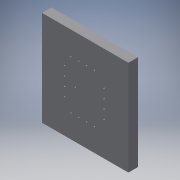
# Autodesk Inventor part: Trasera
Saved by Autodesk Inventor 2017 (Build 210142000, 142)
## iProperties
Created: 2021-02-12
Part Number: Trasera
Material: Generic
Document SubType Name: Modeling
Designer: USUARIO
Density: 1 g/cm^3
Appearance: Default
Author: USUARIO
Autodesk Inventor part; units mm, degrees
ref_plane "YZ Plane" through (0, 0, 0) normal (1, 0, 0) x (0, 1, 0)
ref_plane "XZ Plane" through (0, 0, 0) normal (0, 1, 0) x (-1, 0, 0)
ref_plane "XY Plane" through (0, 0, 0) normal (0, 0, 1) x (1, 0, 0)
sketch "Sketch1" plane through (0, 0, 0) normal (0, 1, 0) x (-1, 0, 0)
  line L0 (0, 0) -> (460, 0)
  line L1 (460, 0) -> (460, -507)
  line L2 (460, -507) -> (0, -507)
  line L3 (0, -507) -> (0, 0)
  dimension "d0" = 460
  dimension "d1" = 507
  constraints: 8 end point, 2 parallel, 1 horizontal, 1 perpendicular
  measures "d0" distance of L1.end L2.end
  measures "d1" distance of L0.end L1.end
extrude "Extrusion1" add sketch "Sketch1" along normal blind 50.8
sketch "Sketch2" plane through (0, 50.8, 0) normal (0, 1, 0) x (1, 0, 0)
  circle A0 centre (-285, 253.5) radius 5
  line L0 (0, 507) -> (-460, 507) projected
  line L1 (0, 0) -> (0, 507) projected
  line L2 (-460, 507) -> (-460, 0) projected
  dimension "d4" = 10
  dimension "d10" = 253.5
  dimension "d11" = 175
  constraints: 1 centre point
  measures "d4" diameter of A0
  measures "d10" distance from line of L0 A0.centre
  measures "d11" distance from line of L2 A0.centre
extrude "Extrusion2" cut sketch "Sketch2" against normal blind 50.8
sketch "Sketch3" plane through (0, 50.8, 0) normal (0, 1, 0) x (1, 0, 0)
  circle A0 centre (-182.3, 123.5) radius 5
  line L0 (0, 0) -> (0, 507) projected
  line L1 (-460, 0) -> (0, 0) projected
  circle A1 centre (-224.3, 123.5) radius 5
  circle A2 centre (-266.3, 123.5) radius 5
  circle A3 centre (-308.3, 123.5) radius 5
  dimension "d12" = 10
  dimension "d13" = 182.3
  dimension "d14" = 123.5
  dimension "d20" = 42
  constraints: 4 centre point, 1 horizontal, 6 other
  measures "d12" diameter of A0
  measures "d13" distance from line of A0.centre L0
  measures "d14" distance from line of A0.centre L1
  measures "d20" distance of A0.centre A1.centre
extrude "Extrusion3" cut sketch "Sketch3" against normal blind 50.8
sketch "Sketch4" plane through (0, 50.8, 0) normal (0, 1, 0) x (1, 0, 0)
  circle A0 centre (-182.3, 383.5) radius 5
  line L0 (0, 0) -> (0, 507) projected
  line L1 (0, 507) -> (-460, 507) projected
  circle A1 centre (-224.3, 383.5) radius 5
  circle A2 centre (-266.3, 383.5) radius 5
  circle A3 centre (-308.3, 383.5) radius 5
  dimension "d24" = 10
  dimension "d25" = 182.3
  dimension "d26" = 123.5
  dimension "d32" = 42
  constraints: 4 centre point, 1 horizontal, 6 other
  measures "d24" diameter of A0
  measures "d25" distance from line of A0.centre L0
  measures "d26" distance from line of A0.centre L1
  measures "d32" distance of A0.centre A1.centre
extrude "Extrusion4" cut sketch "Sketch4" against normal blind 50.8
sketch "Sketch5" plane through (0, 50.8, 0) normal (0, 1, 0) x (1, 0, 0)
  circle A0 centre (-341.5, 181.2) radius 5
  line L0 (-460, 507) -> (-460, 0) projected
  line L1 (-460, 0) -> (0, 0) projected
  circle A1 centre (-131.3, 181.2) radius 5
  line L2 (0, 0) -> (0, 507) projected
  circle A2 centre (-341.5, 229.2) radius 5
  circle A3 centre (-131.3, 229.2) radius 5
  circle A4 centre (-341.5, 277.2) radius 5
  circle A5 centre (-131.3, 277.2) radius 5
  circle A6 centre (-341.5, 325.2) radius 5
  circle A7 centre (-131.3, 325.2) radius 5
  dimension "d36" = 10
  dimension "d37" = 118.5
  dimension "d38" = 181.2
  dimension "d39" = 10
  dimension "d40" = 181.2
  dimension "d41" = 131.3
  dimension "d47" = 48
  constraints: 8 centre point, 1 vertical, 12 other
  measures "d36" diameter of A0
  measures "d37" distance from line of A0.centre L0
  measures "d38" distance from line of A0.centre L1
  measures "d39" diameter of A1
  measures "d40" distance from line of A1.centre L1
  measures "d41" distance from line of A1.centre L2
  measures "d47" distance of A0.centre A2.centre
extrude "Extrusion5" cut sketch "Sketch5" against normal blind 50.8
body "Solid1"
